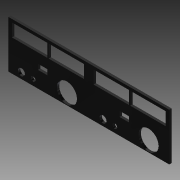
# Autodesk Inventor part: NavCom_mask
Saved by Autodesk Inventor 2014 (Build 180170000, 170)
## iProperties
Created: 2017-02-12
Part Number: NavCom_mask
Material: Všeobecné
Document SubType Name: Modeling
Designer: N
Mass: 14.3892 g
Surface Area: 142.322 cm^2
Volume: 14.3892 cm^3
Density: 1 g/cm^3
Appearance: Výchozí
Author: N
Autodesk Inventor part; units mm, degrees
ref_plane "YZ Plane" through (0, 0, 0) normal (1, 0, 0) x (0, 1, 0)
ref_plane "XZ Plane" through (0, 0, 0) normal (0, 1, 0) x (-1, 0, 0)
ref_plane "XY Plane" through (0, 0, 0) normal (0, 0, 1) x (1, 0, 0)
sketch "Náčrt1" plane through (0, 0, 0) normal (0, 0, 1) x (1, 0, 0)
  point P0 (0, 0)
sketch "Náčrt2" plane through (0, 0, 0) normal (0, 0, 1) x (1, 0, 0)
  line L0 (130.81, 47.627) -> (168.91, 47.625)
  line L1 (168.91, 47.625) -> (168.91, 33.655)
  line L2 (168.91, 33.655) -> (130.81, 33.655)
  line L3 (130.81, 33.655) -> (130.81, 47.627)
  line L4 (3.81, 47.625) -> (41.91, 47.625)
  line L5 (41.91, 47.625) -> (41.91, 33.655)
  line L6 (41.91, 33.655) -> (3.81, 33.655)
  line L7 (3.81, 33.655) -> (3.81, 47.625)
  line L8 (43.18, 47.625) -> (81.28, 47.625)
  line L9 (81.28, 47.625) -> (81.28, 33.655)
  line L10 (81.28, 33.655) -> (43.18, 33.655)
  line L11 (43.18, 33.655) -> (43.18, 47.625)
  line L12 (91.44, 47.625) -> (129.54, 47.625)
  line L13 (129.54, 47.625) -> (129.54, 33.655)
  line L14 (129.54, 33.655) -> (91.44, 33.655)
  line L15 (91.44, 33.655) -> (91.44, 47.625)
  circle A0 centre (26.67, 6.35) radius 2.54
  circle A1 centre (13.97, 6.35) radius 3.81
  circle A2 centre (62.865, 11.43) radius 10.795
  circle A3 centre (114.3, 6.35) radius 2.54
  circle A4 centre (101.6, 6.35) radius 3.81
  circle A5 centre (150.495, 11.43) radius 10.795
  line L16 (31.75, 23.1775) -> (41.91, 23.1775)
  line L17 (41.91, 23.1775) -> (41.91, 17.4625)
  line L18 (41.91, 17.4625) -> (31.75, 17.4625)
  line L19 (31.75, 17.4625) -> (31.75, 23.1775)
  line L20 (119.38, 23.1775) -> (129.54, 23.1775)
  line L21 (129.54, 23.1775) -> (129.54, 17.4625)
  line L22 (129.54, 17.4625) -> (119.38, 17.4625)
  line L23 (119.38, 17.4625) -> (119.38, 23.1775)
  line L24 (0, 50.8) -> (172.72, 50.8)
  line L25 (172.72, 50.8) -> (172.72, 0)
  line L26 (172.72, 0) -> (0, 0)
  line L27 (0, 0) -> (0, 50.8)
  constraints: 56 end point, 6 centre point
extrude "Vysunutí1" add sketch "Náčrt2" along normal blind 2.54
